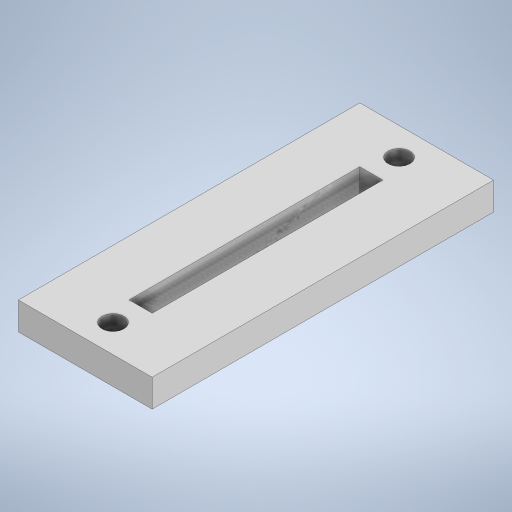
# Autodesk Inventor part: sotenedor
Saved by Autodesk Inventor 2023 (Build 270158000, 158)
## iProperties
Created: 2023-06-06
Part Number: sotenedor
Material: Genérico
Document SubType Name: Modeling
Designer: sergi
Density: 1 g/cm^3
Appearance: Valor por defecto
Author: sergi
Autodesk Inventor part; units mm, degrees
ref_plane "YZ Plane" through (0, 0, 0) normal (1, 0, 0) x (0, 1, 0)
ref_plane "XZ Plane" through (0, 0, 0) normal (0, 1, 0) x (-1, 0, 0)
ref_plane "XY Plane" through (0, 0, 0) normal (0, 0, 1) x (1, 0, 0)
sketch "Boceto1" plane through (0, 0, 0) normal (0, 1, 0) x (-1, 0, 0)
  line L0 (-14.5, -37) -> (14.5, -37)
  line L1 (14.5, -37) -> (14.5, 37)
  line L2 (14.5, 37) -> (-14.5, 37)
  line L3 (-14.5, 37) -> (-14.5, -37)
  line L4 (-14.5, -37) -> (14.5, 37) construction
  line L5 (14.5, -37) -> (-14.5, 37) construction
  line L6 (-2.5, -25) -> (2.5, -25)
  line L7 (2.5, -25) -> (2.5, 25)
  line L8 (2.5, 25) -> (-2.5, 25)
  line L9 (-2.5, 25) -> (-2.5, -25)
  line L10 (-2.5, -25) -> (2.5, 25) construction
  line L11 (2.5, -25) -> (-2.5, 25) construction
  point P0 (0, 0)
  dimension "d2" = 5
  dimension "d3" = 50
  dimension "d4" = 12
  dimension "d5" = 12
  constraints: 24 end point, 4 midpoint, 4 parallel, 2 horizontal, 2 perpendicular
  measures "d2" distance of L8.end L7.end
  measures "d3" distance of L6.end L7.end
  measures "d4" distance between parallel lines of L1 L7
  measures "d5" distance between parallel lines of L0 L6
extrude "Extrusión1" add sketch "Boceto1" along normal blind 6
sketch "Boceto2" plane through (0, 6, 0) normal (0, 1, 0) x (1, 0, 0)
  circle A0 centre (0, -31) radius 2.3812
  line L0 (-14.5, -37) -> (14.5, -37) projected
  point P0 (0, 0)
  dimension "d8" = 4.7625
  dimension "d9" = 6
  constraints: 1 centre point, 1 vertical alignment
  measures "d8" diameter of A0
  measures "d9" distance from line of A0.centre L0
extrude "Extrusión2" cut sketch "Boceto2" against normal through all
mirror "Simetría1" about plane through (0, 0, 0) normal (0, 0, 1) of "Extrusión2"
